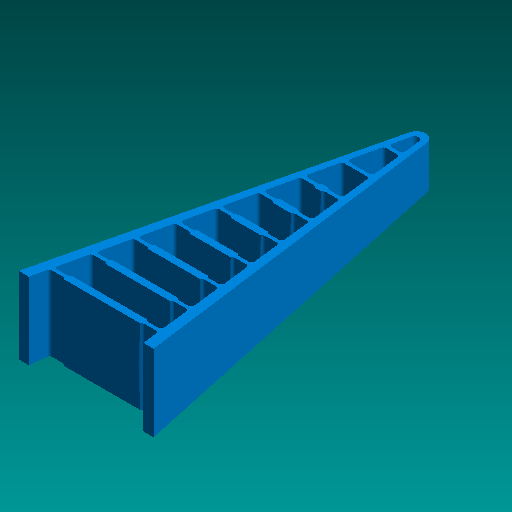
# Autodesk Inventor part: 3998964 DHAS-GF-80-U-BU
Saved by Autodesk Inventor 2020.3 (Build 243373000, 373)
## iProperties
Part Number: 3998964 DHAS-GF-80-U-BU
Material: Generic
Catalog Web Link: www.cadenas.de
Description: DHAS-GF-Adaptive Gripper Finger
Vendor: FESTO
Document SubType Name: Modeling
Designer: partserver
Manufacturer: FESTO
Mass: 13 g
Surface Area: 129.078 cm^2
Volume: 11.9169 cm^3
Density: 1 g/cm^3
Appearance: PSOLRGB-0-153-255
Category: PARTsolutions
Company: FESTO
PSOL_IDENT_0: {$CADENAS_DATA\23d-libs\festo\parts\d\dhas\dhas_gf.prj},188 {VTYP=3D},{NB=3998964 DHAS-GF-80-U-BU},{
PSOL_IDENT_1: LINA=3998964 DHAS-GF-80-U-BU},{NN=DHAS-GF},{DATE=27.04.2020 13:53:14},{GEOMDATE=30.08.2019 14:47:40}
PSOL_IDENT_2: ,{VERSION=},{LINEID=230},{WBVAR=},{WBNUMERIC=}  {NB=3998964 DHAS-GF-80-U-BU},{LINA=3998964 DHAS-GF-8
PSOL_IDENT_3: 0-U-BU},{KT=DUMMY},{TNR=3998964},{TYP=DHAS-GF-80-U-BU},{L=94.5},{CNSMASSEXACT=0.0130},{B1=21.337}
NB: 3998964 DHAS-GF-80-U-BU
NN: DHAS-GF
NT: Adaptive Gripper Finger
NBSYN: $TNR. $TYP.
LINA: 3998964 DHAS-GF-80-U-BU
CATALOG: Festo
TNR: 3998964
TYP: DHAS-GF-80-U-BU
L: 94.5
CNSMASSEXACT: 0.013
SUPPLIER: FESTO
ARTICLENO: 3998964 DHAS-GF-80-U-BU
BOMINFO: 3998964 DHAS-GF-80-U-BU
CREATOR: CADENAS GmbH
Title: 3998964 DHAS-GF-80-U-BU
Author: Cadenas PARTsolutions
Comments: Adaptive Gripper Finger
Autodesk Inventor part; units mm, degrees
ref_plane "YZ Plane" through (0, 0, 0) normal (1, 0, 0) x (0, 1, 0)
ref_plane "XZ Plane" through (0, 0, 0) normal (0, 1, 0) x (-1, 0, 0)
ref_plane "XY Plane" through (0, 0, 0) normal (0, 0, 1) x (1, 0, 0)
sketch "Sketch_1" plane through (0, 0, 0) normal (0, 0, 1) x (1, 0, 0)
  line L0 (-18.761, 0) -> (-15.92, 0)
  line L1 (-15.92, 0) -> (-15.218, 4.3281)
  arc A0 (-14.4283, 5) -> (-15.218, 4.3281) centre (-14.4283, 4.2) ccw
  line L2 (-14.4283, 5) -> (-11.3604, 5)
  arc A1 (-10.795, 4.766) -> (-11.3604, 5) centre (-11.3604, 4.2) ccw
  line L3 (-10.795, 4.766) -> (-10.582, 4.552)
  arc A2 (-10.582, 4.552) -> (-10.0166, 4.318) centre (-10.0166, 5.118) ccw
  line L4 (-10.0166, 4.318) -> (10.0166, 4.318)
  arc A3 (10.0166, 4.318) -> (10.582, 4.552) centre (10.0166, 5.118) ccw
  line L5 (10.582, 4.552) -> (10.795, 4.766)
  arc A4 (11.3604, 5) -> (10.795, 4.766) centre (11.3604, 4.2) ccw
  line L6 (11.3604, 5) -> (14.4283, 5)
  arc A5 (15.218, 4.3281) -> (14.4283, 5) centre (14.4283, 4.2) ccw
  line L7 (15.218, 4.3281) -> (15.92, 0)
  line L8 (15.92, 0) -> (18.761, 0)
  line L9 (18.761, 0) -> (2.462, 92.4341)
  arc A6 (2.462, 92.4341) -> (-2.462, 92.4341) centre (0, 91.9998) ccw
  line L10 (-2.462, 92.4341) -> (-18.761, 0)
  arc A7 (-1.833, 86.928) -> (-1.0433, 86) centre (-1.0433, 86.8) ccw
  line L11 (-1.0433, 86) -> (1.0433, 86)
  arc A8 (1.0433, 86) -> (1.833, 86.928) centre (1.0433, 86.8) ccw
  line L12 (1.833, 86.928) -> (1.066, 91.66)
  arc A9 (1.066, 91.66) -> (0, 92.567) centre (0.0085, 91.497) ccw
  arc A10 (0, 92.567) -> (-1.066, 91.66) centre (-0.0085, 91.497) ccw
  line L13 (-1.066, 91.66) -> (-1.833, 86.928)
  arc A11 (-3.454, 76.928) -> (-2.6643, 76) centre (-2.6643, 76.8) ccw
  line L14 (-2.6643, 76) -> (2.6643, 76)
  arc A12 (2.6643, 76) -> (3.454, 76.928) centre (2.6643, 76.8) ccw
  line L15 (3.454, 76.928) -> (2.255, 84.328)
  arc A13 (2.255, 84.328) -> (1.4653, 85) centre (1.4653, 84.2) ccw
  line L16 (1.4653, 85) -> (-1.4653, 85)
  arc A14 (-1.4653, 85) -> (-2.255, 84.328) centre (-1.4653, 84.2) ccw
  line L17 (-2.255, 84.328) -> (-3.454, 76.928)
  arc A15 (-5.074, 66.928) -> (-4.2843, 66) centre (-4.2843, 66.8) ccw
  line L18 (-4.2843, 66) -> (-1.6914, 66)
  arc A16 (-1.6914, 66) -> (-1.1257, 66.2343) centre (-1.6914, 66.8) ccw
  line L19 (-1.1257, 66.2343) -> (-0.7133, 66.6467)
  arc A17 (-0.1476, 66.881) -> (-0.7133, 66.6467) centre (-0.1476, 66.081) ccw
  line L20 (-0.1476, 66.881) -> (0.1476, 66.881)
  arc A18 (0.7133, 66.6467) -> (0.1476, 66.881) centre (0.1476, 66.081) ccw
  line L21 (0.7133, 66.6467) -> (1.1257, 66.2343)
  arc A19 (1.1257, 66.2343) -> (1.6914, 66) centre (1.6914, 66.8) ccw
  line L22 (1.6914, 66) -> (4.2843, 66)
  arc A20 (4.2843, 66) -> (5.074, 66.928) centre (4.2843, 66.8) ccw
  line L23 (5.074, 66.928) -> (3.875, 74.328)
  arc A21 (3.875, 74.328) -> (3.0853, 75) centre (3.0853, 74.2) ccw
  line L24 (3.0853, 75) -> (-3.0853, 75)
  arc A22 (-3.0853, 75) -> (-3.875, 74.328) centre (-3.0853, 74.2) ccw
  line L25 (-3.875, 74.328) -> (-5.074, 66.928)
  arc A23 (-6.695, 56.928) -> (-5.9053, 56) centre (-5.9053, 56.8) ccw
  line L26 (-5.9053, 56) -> (-3.3024, 56)
  arc A24 (-3.3024, 56) -> (-2.736, 56.235) centre (-3.3024, 56.8) ccw
  line L27 (-2.736, 56.235) -> (-2.2973, 56.6752)
  arc A25 (-1.7316, 56.91) -> (-2.2973, 56.6752) centre (-1.7311, 56.11) ccw
  line L28 (-1.7316, 56.91) -> (1.7316, 56.91)
  arc A26 (2.2973, 56.6752) -> (1.7316, 56.91) centre (1.7311, 56.11) ccw
  line L29 (2.2973, 56.6752) -> (2.737, 56.234)
  arc A27 (2.737, 56.234) -> (3.3024, 56) centre (3.3024, 56.8) ccw
  line L30 (3.3024, 56) -> (5.9053, 56)
  arc A28 (5.9053, 56) -> (6.695, 56.928) centre (5.9053, 56.8) ccw
  line L31 (6.695, 56.928) -> (5.496, 64.328)
  arc A29 (5.496, 64.328) -> (4.7063, 65) centre (4.7063, 64.2) ccw
  line L32 (4.7063, 65) -> (1.6914, 65)
  arc A30 (1.6914, 65) -> (1.126, 64.766) centre (1.6914, 64.2) ccw
  line L33 (1.126, 64.766) -> (0.966, 64.605)
  arc A31 (0.4006, 64.371) -> (0.966, 64.605) centre (0.4006, 65.171) ccw
  line L34 (0.4006, 64.371) -> (-0.4006, 64.371)
  arc A32 (-0.966, 64.605) -> (-0.4006, 64.371) centre (-0.4006, 65.171) ccw
  line L35 (-0.966, 64.605) -> (-1.126, 64.766)
  arc A33 (-1.126, 64.766) -> (-1.6914, 65) centre (-1.6914, 64.2) ccw
  line L36 (-1.6914, 65) -> (-4.7063, 65)
  arc A34 (-4.7063, 65) -> (-5.496, 64.328) centre (-4.7063, 64.2) ccw
  line L37 (-5.496, 64.328) -> (-6.695, 56.928)
  arc A35 (-8.315, 46.928) -> (-7.5253, 46) centre (-7.5253, 46.8) ccw
  line L38 (-7.5253, 46) -> (-4.9144, 46)
  arc A36 (-4.9144, 46) -> (-4.3487, 46.2343) centre (-4.9144, 46.8) ccw
  line L39 (-4.3487, 46.2343) -> (-3.8813, 46.7017)
  arc A37 (-3.3156, 46.936) -> (-3.8813, 46.7017) centre (-3.3156, 46.136) ccw
  line L40 (-3.3156, 46.936) -> (3.3156, 46.936)
  arc A38 (3.8813, 46.7017) -> (3.3156, 46.936) centre (3.3156, 46.136) ccw
  line L41 (3.8813, 46.7017) -> (4.3487, 46.2343)
  arc A39 (4.3487, 46.2343) -> (4.9144, 46) centre (4.9144, 46.8) ccw
  line L42 (4.9144, 46) -> (7.5253, 46)
  arc A40 (7.5253, 46) -> (8.315, 46.928) centre (7.5253, 46.8) ccw
  line L43 (8.315, 46.928) -> (7.116, 54.328)
  arc A41 (7.116, 54.328) -> (6.3263, 55) centre (6.3263, 54.2) ccw
  line L44 (6.3263, 55) -> (3.3024, 55)
  arc A42 (3.3024, 55) -> (2.737, 54.766) centre (3.3024, 54.2) ccw
  line L45 (2.737, 54.766) -> (2.569, 54.595)
  arc A43 (2.0026, 54.36) -> (2.569, 54.595) centre (2.0026, 55.16) ccw
  line L46 (2.0026, 54.36) -> (-2.0026, 54.36)
  arc A44 (-2.569, 54.595) -> (-2.0026, 54.36) centre (-2.0026, 55.16) ccw
  line L47 (-2.569, 54.595) -> (-2.737, 54.766)
  arc A45 (-2.737, 54.766) -> (-3.3024, 55) centre (-3.3024, 54.2) ccw
  line L48 (-3.3024, 55) -> (-6.3263, 55)
  arc A46 (-6.3263, 55) -> (-7.116, 54.328) centre (-6.3263, 54.2) ccw
  line L49 (-7.116, 54.328) -> (-8.315, 46.928)
  arc A47 (-9.936, 36.928) -> (-9.1463, 36) centre (-9.1463, 36.8) ccw
  line L50 (-9.1463, 36) -> (-6.5264, 36)
  arc A48 (-6.5264, 36) -> (-5.961, 36.234) centre (-6.5264, 36.8) ccw
  line L51 (-5.961, 36.234) -> (-5.4719, 36.7311)
  arc A49 (-4.9016, 36.97) -> (-5.4719, 36.7311) centre (-4.9016, 36.17) ccw
  line L52 (-4.9016, 36.97) -> (4.9016, 36.97)
  arc A50 (5.4719, 36.7311) -> (4.9016, 36.97) centre (4.9016, 36.17) ccw
  line L53 (5.4719, 36.7311) -> (5.961, 36.234)
  arc A51 (5.961, 36.234) -> (6.5264, 36) centre (6.5264, 36.8) ccw
  line L54 (6.5264, 36) -> (9.1463, 36)
  arc A52 (9.1463, 36) -> (9.936, 36.928) centre (9.1463, 36.8) ccw
  line L55 (9.936, 36.928) -> (8.737, 44.328)
  arc A53 (8.737, 44.328) -> (7.9473, 45) centre (7.9473, 44.2) ccw
  line L56 (7.9473, 45) -> (4.9144, 45)
  arc A54 (4.9144, 45) -> (4.3487, 44.7657) centre (4.9144, 44.2) ccw
  line L57 (4.3487, 44.7657) -> (4.1703, 44.5873)
  arc A55 (3.6046, 44.353) -> (4.1703, 44.5873) centre (3.6046, 45.153) ccw
  line L58 (3.6046, 44.353) -> (-3.6046, 44.353)
  arc A56 (-4.1703, 44.5873) -> (-3.6046, 44.353) centre (-3.6046, 45.153) ccw
  line L59 (-4.1703, 44.5873) -> (-4.3487, 44.7657)
  arc A57 (-4.3487, 44.7657) -> (-4.9144, 45) centre (-4.9144, 44.2) ccw
  line L60 (-4.9144, 45) -> (-7.9473, 45)
  arc A58 (-7.9473, 45) -> (-8.737, 44.328) centre (-7.9473, 44.2) ccw
  line L61 (-8.737, 44.328) -> (-9.936, 36.928)
  arc A59 (-11.556, 26.928) -> (-10.7663, 26) centre (-10.7663, 26.8) ccw
  line L62 (-10.7663, 26) -> (-8.1374, 26)
  arc A60 (-8.1374, 26) -> (-7.5717, 26.2343) centre (-8.1374, 26.8) ccw
  line L63 (-7.5717, 26.2343) -> (-7.0513, 26.7547)
  arc A61 (-6.4856, 26.989) -> (-7.0513, 26.7547) centre (-6.4856, 26.189) ccw
  line L64 (-6.4856, 26.989) -> (6.4856, 26.989)
  arc A62 (7.0513, 26.7547) -> (6.4856, 26.989) centre (6.4856, 26.189) ccw
  line L65 (7.0513, 26.7547) -> (7.5717, 26.2343)
  arc A63 (7.5717, 26.2343) -> (8.1374, 26) centre (8.1374, 26.8) ccw
  line L66 (8.1374, 26) -> (10.7663, 26)
  arc A64 (10.7663, 26) -> (11.556, 26.928) centre (10.7663, 26.8) ccw
  line L67 (11.556, 26.928) -> (10.357, 34.328)
  arc A65 (10.357, 34.328) -> (9.5673, 35) centre (9.5673, 34.2) ccw
  line L68 (9.5673, 35) -> (6.5264, 35)
  arc A66 (6.5264, 35) -> (5.9607, 34.7657) centre (6.5264, 34.2) ccw
  line L69 (5.9607, 34.7657) -> (5.7733, 34.5783)
  arc A67 (5.2076, 34.344) -> (5.7733, 34.5783) centre (5.2076, 35.144) ccw
  line L70 (5.2076, 34.344) -> (-5.2076, 34.344)
  arc A68 (-5.7733, 34.5783) -> (-5.2076, 34.344) centre (-5.2076, 35.144) ccw
  line L71 (-5.7733, 34.5783) -> (-5.9607, 34.7657)
  arc A69 (-5.9607, 34.7657) -> (-6.5264, 35) centre (-6.5264, 34.2) ccw
  line L72 (-6.5264, 35) -> (-9.5673, 35)
  arc A70 (-9.5673, 35) -> (-10.357, 34.328) centre (-9.5673, 34.2) ccw
  line L73 (-10.357, 34.328) -> (-11.556, 26.928)
  arc A71 (-13.177, 16.9281) -> (-12.3873, 16) centre (-12.3873, 16.8) ccw
  line L74 (-12.3873, 16) -> (-9.7494, 16)
  arc A72 (-9.7494, 16) -> (-9.1837, 16.2343) centre (-9.7494, 16.8) ccw
  line L75 (-9.1837, 16.2343) -> (-8.6373, 16.7807)
  arc A73 (-8.0716, 17.015) -> (-8.6373, 16.7807) centre (-8.0716, 16.215) ccw
  line L76 (-8.0716, 17.015) -> (8.0716, 17.015)
  arc A74 (8.6373, 16.7807) -> (8.0716, 17.015) centre (8.0716, 16.215) ccw
  line L77 (8.6373, 16.7807) -> (9.1837, 16.2343)
  arc A75 (9.1837, 16.2343) -> (9.7494, 16) centre (9.7494, 16.8) ccw
  line L78 (9.7494, 16) -> (12.3873, 16)
  arc A76 (12.3873, 16) -> (13.177, 16.9281) centre (12.3873, 16.8) ccw
  line L79 (13.177, 16.9281) -> (11.977, 24.3281)
  arc A77 (11.977, 24.3281) -> (11.1873, 25) centre (11.1873, 24.2) ccw
  line L80 (11.1873, 25) -> (8.1374, 25)
  arc A78 (8.1374, 25) -> (7.5717, 24.7657) centre (8.1374, 24.2) ccw
  line L81 (7.5717, 24.7657) -> (7.3753, 24.5693)
  arc A79 (6.8096, 24.335) -> (7.3753, 24.5693) centre (6.8096, 25.135) ccw
  line L82 (6.8096, 24.335) -> (-6.8096, 24.335)
  arc A80 (-7.3753, 24.5693) -> (-6.8096, 24.335) centre (-6.8096, 25.135) ccw
  line L83 (-7.3753, 24.5693) -> (-7.5717, 24.7657)
  arc A81 (-7.5717, 24.7657) -> (-8.1374, 25) centre (-8.1374, 24.2) ccw
  line L84 (-8.1374, 25) -> (-11.1873, 25)
  arc A82 (-11.1873, 25) -> (-11.977, 24.3281) centre (-11.1873, 24.2) ccw
  line L85 (-11.977, 24.3281) -> (-13.177, 16.9281)
  arc A83 (-14.797, 6.928) -> (-14.0073, 6) centre (-14.0073, 6.8) ccw
  line L86 (-14.0073, 6) -> (-11.3604, 6)
  arc A84 (-11.3604, 6) -> (-10.7942, 6.2348) centre (-11.3604, 6.8) ccw
  line L87 (-10.7942, 6.2348) -> (-10.2228, 6.8072)
  arc A85 (-9.6566, 7.042) -> (-10.2228, 6.8072) centre (-9.6566, 6.242) ccw
  line L88 (-9.6566, 7.042) -> (9.6566, 7.042)
  arc A86 (10.2228, 6.8072) -> (9.6566, 7.042) centre (9.6566, 6.242) ccw
  line L89 (10.2228, 6.8072) -> (10.7942, 6.2348)
  arc A87 (10.7942, 6.2348) -> (11.3604, 6) centre (11.3604, 6.8) ccw
  line L90 (11.3604, 6) -> (14.0073, 6)
  arc A88 (14.0073, 6) -> (14.797, 6.928) centre (14.0073, 6.8) ccw
  line L91 (14.797, 6.928) -> (13.598, 14.328)
  arc A89 (13.598, 14.328) -> (12.8083, 15) centre (12.8083, 14.2) ccw
  line L92 (12.8083, 15) -> (9.7494, 15)
  arc A90 (9.7494, 15) -> (9.1837, 14.7657) centre (9.7494, 14.2) ccw
  line L93 (9.1837, 14.7657) -> (8.9793, 14.5613)
  arc A91 (8.4136, 14.327) -> (8.9793, 14.5613) centre (8.4136, 15.127) ccw
  line L94 (8.4136, 14.327) -> (-8.4136, 14.327)
  arc A92 (-8.9793, 14.5613) -> (-8.4136, 14.327) centre (-8.4136, 15.127) ccw
  line L95 (-8.9793, 14.5613) -> (-9.1837, 14.7657)
  arc A93 (-9.1837, 14.7657) -> (-9.7494, 15) centre (-9.7494, 14.2) ccw
  line L96 (-9.7494, 15) -> (-12.8083, 15)
  arc A94 (-12.8083, 15) -> (-13.598, 14.328) centre (-12.8083, 14.2) ccw
  line L97 (-13.598, 14.328) -> (-14.797, 6.928)
  constraints: 196 end point, 190 point on circle, 95 centre point
extrude "Extrusion1" add sketch "Sketch_1" along normal mid plane 31.337
sketch "Sketch_2" plane through (0, 0, 0) normal (1, 0, 0) x (0, 1, 0)
  line L0 (104.5, 21.337) -> (-10, 21.337)
  line L1 (-10, 21.337) -> (-10, -21.337)
  line L2 (-10, -21.337) -> (104.5, -21.337)
  line L3 (104.5, -21.337) -> (104.5, 21.337)
  line L4 (0, 10.6685) -> (0, -10.6685)
  line L5 (0, -10.6685) -> (94.5, -5.8813)
  line L6 (94.5, -5.8813) -> (94.5, 5.8813)
  line L7 (94.5, 5.8813) -> (0, 10.6685)
  constraints: 16 end point
extrude "Extrusion2" cut sketch "Sketch_2" along normal mid plane 70
sketch "Sketch_3" plane through (0, 0, 0) normal (1, 0, 0) x (0, 1, 0)
  line L0 (9, 20) -> (4, 20)
  line L1 (4, 20) -> (4, -20)
  line L2 (4, -20) -> (9, -20)
  line L3 (9, -20) -> (9, 20)
  line L4 (4.5, 10.4405) -> (4.3178, 0)
  line L5 (4.3178, 0) -> (4.5, -10.4405)
  line L6 (4.5, -10.4405) -> (6.5, -10.3392)
  line L7 (6.5, -10.3392) -> (7.0419, 0)
  line L8 (7.0419, 0) -> (6.5, 10.3392)
  line L9 (6.5, 10.3392) -> (4.5, 10.4405)
  constraints: 20 end point
extrude "Extrusion3" cut sketch "Sketch_3" along normal mid plane 24
sketch "Sketch_4" plane through (0, 0, 0) normal (1, 0, 0) x (0, 1, 0)
  line L0 (18, 20) -> (13, 20)
  line L1 (13, 20) -> (13, -20)
  line L2 (13, -20) -> (18, -20)
  line L3 (18, -20) -> (18, 20)
  line L4 (14.5, 9.934) -> (14.3266, 0)
  line L5 (14.3266, 0) -> (14.5, -9.934)
  line L6 (14.5, -9.934) -> (16.5, -9.8326)
  line L7 (16.5, -9.8326) -> (17.0153, 0)
  line L8 (17.0153, 0) -> (16.5, 9.8326)
  line L9 (16.5, 9.8326) -> (14.5, 9.934)
  constraints: 20 end point
extrude "Extrusion4" cut sketch "Sketch_4" along normal mid plane 20
sketch "Sketch_5" plane through (0, 0, 0) normal (1, 0, 0) x (0, 1, 0)
  line L0 (28, 20) -> (23, 20)
  line L1 (23, 20) -> (23, -20)
  line L2 (23, -20) -> (28, -20)
  line L3 (28, -20) -> (28, 20)
  line L4 (24.5, 9.4274) -> (24.3354, 0)
  line L5 (24.3354, 0) -> (24.5, -9.4274)
  line L6 (24.5, -9.4274) -> (26.5, -9.3261)
  line L7 (26.5, -9.3261) -> (26.9888, 0)
  line L8 (26.9888, 0) -> (26.5, 9.3261)
  line L9 (26.5, 9.3261) -> (24.5, 9.4274)
  constraints: 20 end point
extrude "Extrusion5" cut sketch "Sketch_5" along normal mid plane 18
sketch "Sketch_6" plane through (0, 0, 0) normal (1, 0, 0) x (0, 1, 0)
  line L0 (38, 20) -> (33, 20)
  line L1 (33, 20) -> (33, -20)
  line L2 (33, -20) -> (38, -20)
  line L3 (38, -20) -> (38, 20)
  line L4 (34.5, 8.9208) -> (34.3443, 0)
  line L5 (34.3443, 0) -> (34.5, -8.9208)
  line L6 (34.5, -8.9208) -> (36.5, -8.8195)
  line L7 (36.5, -8.8195) -> (36.9622, 0)
  line L8 (36.9622, 0) -> (36.5, 8.8195)
  line L9 (36.5, 8.8195) -> (34.5, 8.9208)
  constraints: 20 end point
extrude "Extrusion6" cut sketch "Sketch_6" along normal mid plane 16
sketch "Sketch_7" plane through (0, 0, 0) normal (1, 0, 0) x (0, 1, 0)
  line L0 (48, 20) -> (43, 20)
  line L1 (43, 20) -> (43, -20)
  line L2 (43, -20) -> (48, -20)
  line L3 (48, -20) -> (48, 20)
  line L4 (44.5, 8.4142) -> (44.3531, 0)
  line L5 (44.3531, 0) -> (44.5, -8.4142)
  line L6 (44.5, -8.4142) -> (46.5, -8.3129)
  line L7 (46.5, -8.3129) -> (46.9357, 0)
  line L8 (46.9357, 0) -> (46.5, 8.3129)
  line L9 (46.5, 8.3129) -> (44.5, 8.4142)
  constraints: 20 end point
extrude "Extrusion7" cut sketch "Sketch_7" along normal mid plane 14
sketch "Sketch_8" plane through (0, 0, 0) normal (1, 0, 0) x (0, 1, 0)
  line L0 (58, 20) -> (53, 20)
  line L1 (53, 20) -> (53, -20)
  line L2 (53, -20) -> (58, -20)
  line L3 (58, -20) -> (58, 20)
  line L4 (54.5, 7.9076) -> (54.362, 0)
  line L5 (54.362, 0) -> (54.5, -7.9076)
  line L6 (54.5, -7.9076) -> (56.5, -7.8063)
  line L7 (56.5, -7.8063) -> (56.9091, 0)
  line L8 (56.9091, 0) -> (56.5, 7.8063)
  line L9 (56.5, 7.8063) -> (54.5, 7.9076)
  constraints: 20 end point
extrude "Extrusion8" cut sketch "Sketch_8" along normal mid plane 8
sketch "Sketch_9" plane through (0, 0, 0) normal (1, 0, 0) x (0, 1, 0)
  line L0 (68, 20) -> (63, 20)
  line L1 (63, 20) -> (63, -20)
  line L2 (63, -20) -> (68, -20)
  line L3 (68, -20) -> (68, 20)
  line L4 (64.5, 7.4011) -> (64.3708, 0)
  line L5 (64.3708, 0) -> (64.5, -7.4011)
  line L6 (64.5, -7.4011) -> (66.5, -7.2998)
  line L7 (66.5, -7.2998) -> (66.8826, 0)
  line L8 (66.8826, 0) -> (66.5, 7.2998)
  line L9 (66.5, 7.2998) -> (64.5, 7.4011)
  constraints: 20 end point
extrude "Extrusion9" cut sketch "Sketch_9" along normal mid plane 4
body "Solid1"
